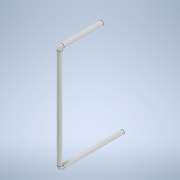
# Autodesk Inventor part: pipe
Saved by Autodesk Inventor 2021 (Build 250183000, 183)
## iProperties
Created: 2021-07-06
Part Number: pipe
Material: Generic
Document SubType Name: Modeling
Designer: HP
Density: 1 g/cm^3
Appearance: Default
Author: HP
Autodesk Inventor part; units mm, degrees
ref_plane "YZ Plane" through (0, 0, 0) normal (1, 0, 0) x (0, 1, 0)
ref_plane "XY Plane" through (0, 0, 0) normal (0, 0, 1) x (1, 0, 0)
sketch "Sketch1" plane through (0, 0, 0) normal (0, 0, 1) x (1, 0, 0)
  circle A0 centre (-1.5437, 0) radius 100
  point P0 (0, 0)
  dimension "d0" = 200
  constraints: 1 centre point
  measures "d0" diameter of A0
extrude "Extrusion1" add sketch "Sketch1" against normal blind 10000
ref_plane "Work Plane1" through (-1.5437, 100, 0) normal (0, 1, 0) x (-1, 0, 0)
sketch "Sketch2" plane through (-1.5437, 100, 0) normal (0, 1, 0) x (-1, 0, 0)
  line L0 (957.6354, -2000) -> (-1190.1544, -2000)
  line L1 (100, 0) -> (-100, 0) projected
  line L2 (957.6354, -5000) -> (-3348.8895, -5000)
  point P0 (-1.5437, 0)
  dimension "d3" = 2000
  dimension "d4" = 3000
  constraints: 4 end point, 2 horizontal
  measures "d3" distance between parallel lines of L0 L1
  measures "d4" distance between parallel lines of L2 L0
bend part "Bend Part1" radius 25.4 angle 90 line through (-959.1791, 100, -2000) along (1, 0, 0) centre toward (0, 1, 0) moving side (0, 0, 1) both sides no
sketch "Sketch3" plane through (-1.5437, 100, 0) normal (0, 1, 0) x (-1, 0, 0)
  line L0 (2900.7515, -7000) -> (-2448.0978, -7000)
  line L1 (-100, -10000) -> (100, -10000) projected
  point P0 (-1.5437, 0)
  dimension "d7" = 3000
  constraints: 2 end point, 1 horizontal
  measures "d7" distance between parallel lines of L1 L0
bend part "Bend Part2" radius 25.4 angle 90 line through (-2902.2952, 100, -7000) along (1, 0, 0) centre toward (0, 1, 0) moving side (0, 0, 1) both sides no
shell "Shell1" thickness 10 removed faces 1 at (-11.7612, 5158.0703, -8960.1018)
sketch "Sketch4" plane through (-1.5437, 0, -10000) normal (0, 0, -1) x (-1, 0, 0)
  circle A0 centre (0, 0) radius 90 projected
  circle A1 centre (0, 0) radius 375
  point P0 (-1.5437, 0)
  constraints: 1 centre point, 1 coincident
extrude "Extrusion2" cut sketch "Sketch4" against normal blind 1500 contours A0
body "Solid1"
